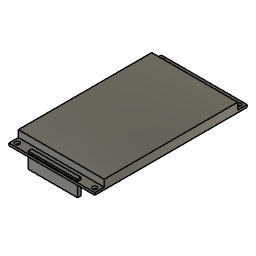
Screen (Autodesk Fusion 360 design; units mm, degrees)
Autodesk Fusion 360 part; units mm, degrees
sketch "Sketch1" plane through (0, 0, 0) normal (0, 0, 1) x (1, 0, 0)
  line L0 (0, 0) -> (60.88, 0)
  line L1 (60.88, 0) -> (60.88, 108)
  line L2 (60.88, 108) -> (0, 108)
  line L3 (0, 108) -> (0, 0)
  circle A0 centre (3, 3) radius 1.6
  circle A1 centre (57.88, 3) radius 1.6
  circle A2 centre (3, 105) radius 1.6
  circle A3 centre (57.88, 105) radius 1.6
  line L4 (0, 101.29) -> (60.88, 101.29)
  line L5 (60.88, 101.29) -> (60.88, 6.72)
  line L6 (60.88, 6.72) -> (0, 6.72)
  line L7 (0, 6.72) -> (0, 101.29)
  dimension "d1" = 60.88
  dimension "d2" = 108
  dimension "d3" = 3.2
  dimension "d6" = 54.88
  dimension "d7" = 102
  dimension "d8" = 3
  dimension "d9" = 3
  dimension "d10" = 60.88
  dimension "d11" = 94.57
  dimension "d12" = 6.71
  constraint horizontal L0
  constraint vertical L1
  constraint horizontal L2
  constraint vertical L3
  constraint coincident L0.start L3.end
  constraint horizontal L4
  constraint vertical L5
  constraint horizontal L6
  constraint vertical L7
  constraint collinear L3 L7
  measures "d1" distance of L0.start L0.end
  measures "d2" distance of L0.start L2.end
  measures "d3" diameter of A0
  measures "d8" distance of L0 A0.centre
  measures "d9" distance of L3 A0.centre
  measures "d10" distance of L4.start L4.end
  measures "d11" distance of L4.start L6.end
  measures "d12" distance of L2 L4
extrude "Extrude1" add sketch "Sketch1" along normal blind 1.6 contours L0 L1 L3 L6 | L1 L2 L3 L4 makes body 1 at (39.32, 102.0648, 0) makes body 2 at (21.56, 5.9419, 0)
extrude "Extrude2" add sketch "Sketch1" along normal blind 6.45 contours L1 L3 L4 L5 L6 L7 bodies 1 2
sketch "Sketch2" plane through (0, 0, 0) normal (0, 0, -1) x (1, 0, 0)
  circle A0 centre (57.88, -3) radius 1.6
  circle A1 centre (3, -3) radius 1.6
  circle A2 centre (57.88, -105) radius 1.6
  circle A3 centre (3, -105) radius 1.6
  line L0 (0, 0) -> (0, -108)
  line L1 (0, -108) -> (60.88, -108)
  line L2 (60.88, -108) -> (60.88, 0)
  line L3 (60.88, 0) -> (0, 0)
  line L4 (17, -63.47) -> (0, -63.47)
  line L5 (0, -63.47) -> (0, -48.47)
  line L6 (0, -48.47) -> (17, -48.47)
  line L7 (17, -48.47) -> (17, -63.47)
  point P0 (0, -55.97)
  dimension "d18" = 17
  dimension "d19" = 15
  dimension "d20" = 52.03
  constraint horizontal L4
  constraint vertical L5
  constraint horizontal L6
  constraint vertical L7
  constraint midpoint L5 P0
  constraint collinear L0 L5
  measures "d18" distance of L4.start L4.end
  measures "d19" distance of L4.start L6.end
  measures "d20" distance of L1 P0
extrude "Extrude3" add sketch "Sketch2" along normal blind 2.2 contours L0 L4 L5 L6 L7 bodies 1
sketch "Sketch3" plane through (0, 0, 1.6) normal (0, 0, 1) x (-1, 0, 0)
  circle A0 centre (-3, -3) radius 1.6
  circle A1 centre (-57.88, -3) radius 1.6
  line L0 (-60.88, -6.72) -> (0, -6.72)
  line L1 (0, -6.72) -> (0, 0)
  line L2 (0, 0) -> (-60.88, 0)
  line L3 (-60.88, 0) -> (-60.88, -6.72)
  line L4 (-12.94, -3.27) -> (-47.94, -3.27)
  line L5 (-47.94, -3.27) -> (-47.94, -0.73)
  line L6 (-47.94, -0.73) -> (-12.94, -0.73)
  line L7 (-12.94, -0.73) -> (-12.94, -3.27)
  point P0 (-30.44, -3.27)
  point P1 (-47.94, -2)
  point P2 (-30.44, 0)
  point P3 (-30.44, -0.73)
  dimension "d23" = 35
  dimension "d24" = 2.54
  dimension "d25" = 2
  constraint horizontal L4
  constraint vertical L5
  constraint horizontal L6
  constraint vertical L7
  constraint midpoint L4 P0
  constraint midpoint L5 P1
  constraint midpoint L2 P2
  constraint midpoint L6 P3
  constraint collinear P0 P2 P3
  measures "d23" distance of L4.start L4.end
  measures "d24" distance of L4.start L6.end
  measures "d25" distance of L2 P1
extrude "Extrude4" add sketch "Sketch3" along normal blind 1.23 and the other way blind 9.94 contours L4 L5 L6 L7 bodies 1
equation "d28 = 11.17 mm - 1.23 mm"
